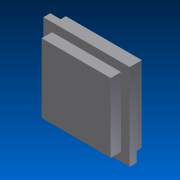
# Autodesk Inventor part: antena_gps
Saved by Autodesk Inventor 2012 (Build 160160000, 160)
## iProperties
Created: 2016-01-19
Part Number: antena_gps
Material: Default
Document SubType Name: Modeling
Designer: Alex Becerra
Mass: 12.6 g
Surface Area: 19.54 cm^2
Volume: 3.902 cm^3
Density: 3.22911 g/cm^3
Author: Alex Becerra
Autodesk Inventor part; units mm, degrees
ref_plane "YZ Plane" through (0, 0, 0) normal (1, 0, 0) x (0, 1, 0)
ref_plane "XZ Plane" through (0, 0, 0) normal (0, 1, 0) x (-1, 0, 0)
ref_plane "XY Plane" through (0, 0, 0) normal (0, 0, 1) x (1, 0, 0)
sketch "Sketch1" plane through (0, 0, 0) normal (0, 0, 1) x (1, 0, 0)
  line L0 (0, 0) -> (25, 0)
  line L1 (25, 0) -> (25, 25)
  line L2 (25, 25) -> (0, 25)
  line L3 (0, 25) -> (0, 0)
  dimension "d0" = 25
  dimension "d1" = 25
  constraints: 8 end point, 2 parallel, 1 horizontal, 1 perpendicular
  measures "d0" distance of L2.end L1.end
  measures "d1" distance of L1.end L0.end
extrude "Extrusion1" add sketch "Sketch1" along normal blind 2
sketch "Sketch2" plane through (0, 0, 2) normal (0, 0, 1) x (1, 0, 0)
  line L0 (0, 0) -> (0, 25) projected
  line L1 (0, 25) -> (25, 25) projected
  line L2 (2.5, 2.5) -> (22.5, 2.5)
  line L3 (22.5, 2.5) -> (22.5, 22.5)
  line L4 (22.5, 22.5) -> (2.5, 22.5)
  line L5 (2.5, 22.5) -> (2.5, 2.5)
  dimension "d4" = 20
  dimension "d5" = 20
  dimension "d6" = 2.5
  dimension "d7" = 2.5
  constraints: 8 end point, 2 parallel, 1 horizontal, 1 perpendicular
  measures "d4" distance of L4.end L3.end
  measures "d5" distance of L3.end L2.end
  measures "d6" distance between parallel lines of L1 L4
  measures "d7" distance between parallel lines of L0 L5
extrude "Extrusion2" add sketch "Sketch2" along normal blind 3
sketch "Sketch3" plane through (0, 0, 0) normal (0, 0, -1) x (-1, 0, 0)
  line L0 (-25, 25) -> (0, 25) projected
  line L1 (-25, 0) -> (-25, 25) projected
  line L2 (-23.5, 23.5) -> (-1.5, 23.5)
  line L3 (-1.5, 23.5) -> (-1.5, 1.5)
  line L4 (-1.5, 1.5) -> (-23.5, 1.5)
  line L5 (-23.5, 1.5) -> (-23.5, 23.5)
  dimension "d10" = 22
  dimension "d11" = 22
  dimension "d12" = 1.5
  dimension "d13" = 1.5
  constraints: 8 end point, 2 parallel, 1 horizontal, 1 perpendicular
  measures "d10" distance of L3.end L4.end
  measures "d11" distance of L2.end L3.end
  measures "d12" distance between parallel lines of L1 L5
  measures "d13" distance between parallel lines of L0 L2
extrude "Extrusion3" add sketch "Sketch3" along normal blind 3
body "Solid1"
